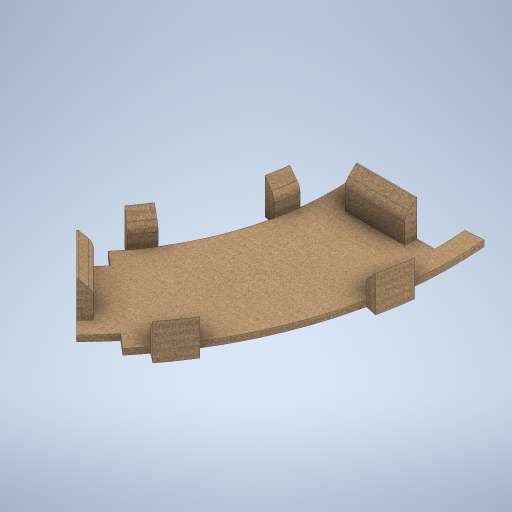
# Autodesk Inventor part: MC Plate
Saved by Autodesk Inventor 2023 (Build 270158000, 158)
## iProperties
Created: 2023-01-27
Part Number: MC Plate
Material: MDF Medium Density Fiberboard
Document SubType Name: Modeling
Designer: cheng
Density: 0.8 g/cm^3
Appearance: Cardboard - Corrugated
Mass: 204.328 g
Surface Area: 611.32 cm^2
Volume: 255.411 cm^3
Author: cheng
Autodesk Inventor part; units mm, degrees
ref_plane "YZ Plane" through (0, 0, 0) normal (1, 0, 0) x (0, 1, 0)
ref_plane "XZ Plane" through (0, 0, 0) normal (0, 1, 0) x (-1, 0, 0)
ref_plane "XY Plane" through (0, 0, 0) normal (0, 0, 1) x (1, 0, 0)
sketch "Sketch1" plane through (0, 0, 0) normal (0, 1, 0) x (-1, 0, 0)
  circle A0 centre (0, 0) radius 215
  circle A1 centre (0, 0) radius 315
  line L0 (0, 0) -> (-315, 0)
  line L1 (0, 0) -> (-222.7386, 222.7386)
  line L2 (0, 0) -> (-313.8013, -27.4541)
  line L3 (0, 0) -> (-241.304, 202.4781)
  circle A2 centre (0, 0) radius 230
  circle A3 centre (0, 0) radius 300
  point P0 (-152.028, 152.028)
  point P1 (-215, 0)
  point P2 (-212.132, 212.132)
  point P3 (-229.8133, 192.8363)
  point P4 (-298.8584, -26.1467)
  point P5 (-300, 0)
  point P6 (-230, 0)
  point P7 (-229.1248, -20.0458)
  point P8 (-214.1819, -18.7385)
  point P9 (-164.6996, 138.1993)
  point P10 (-176.1902, 147.8412)
  point P11 (-162.6346, 162.6346)
  dimension "d1" = 430
  dimension "d2" = 45
  dimension "d31" = 100
  dimension "d47" = 5
  dimension "d48" = 5
  dimension "d49" = 15
  dimension "d50" = 15
  constraints: 8 end point, 4 centre point, 4 coincident, 4 point on circle, 1 horizontal
  measures "d1" diameter of A0
  measures "d2" angle of L0 L1
  measures "d31" radial gap between concentric circles of A0 A1
  measures "d47" angle of L2 L0
  measures "d48" angle of L3 L1
  measures "d49" radial gap between concentric circles of A0 A2
  measures "d50" radial gap between concentric circles of A3 A1
extrude "Extrusion1" add sketch "Sketch1" along normal blind 5 contours L2 A2 L0 A0 | A0 L0 A2 L3 | A2 L3 A3 L1 | A2 L0 A3 L3 | L2 A1 L0 A3 | A3 L0 A1 L3
sketch "Sketch2" plane through (0, 0, 0) normal (0, 1, 0) x (1, 0, 0)
  circle A0 centre (0, 0) radius 205
  circle A1 centre (0, 0) radius 215
  circle A2 centre (0, 0) radius 315
  circle A3 centre (0, 0) radius 325
  line L0 (0, 0) -> (259.5565, -195.5899)
  line L1 (0, 0) -> (275.6156, -172.2238)
  line L2 (0, 0) -> (317.898, -67.5713)
  line L3 (0, 0) -> (322.5775, -39.6075)
  line L4 (300, 0) -> (230, 0) projected
  point P0 (315, 0)
  point P1 (215, 0)
  point P2 (312.652, -38.3888)
  point P3 (308.1165, -65.4922)
  point P4 (213.3974, -26.2019)
  point P5 (203.472, -24.9832)
  point P6 (200.5203, -42.6219)
  point P7 (210.3017, -44.701)
  point P8 (267.1352, -166.9246)
  point P9 (251.5702, -189.5717)
  point P10 (182.3303, -113.9326)
  point P11 (173.8499, -108.6334)
  point P12 (163.7203, -123.3721)
  point P13 (171.7066, -129.3902)
  dimension "d5" = 410
  dimension "d6" = 10
  dimension "d7" = 100
  dimension "d8" = 10
  dimension "d9" = 7
  dimension "d10" = 5
  dimension "d11" = 20
  dimension "d12" = 5
  constraints: 8 end point, 4 centre point, 4 coincident, 4 point on circle
  measures "d5" diameter of A0
  measures "d6" radial gap between concentric circles of A0 A1
  measures "d7" radial gap between concentric circles of A2 A1
  measures "d8" radial gap between concentric circles of A2 A3
  measures "d9" angle of L3 L4
  measures "d10" angle of L2 L3
  measures "d11" angle of L1 L2
  measures "d12" angle of L0 L1
extrude "Extrusion2" add sketch "Sketch2" along normal blind 30 contours A0 L1 A1 L0 | L3 A1 L2 A0 | A2 L1 A3 L0 | L3 A3 L2 A2
chamfer "Chamfer1" distance 10 angle 45 4 edges at (177.1871, 30, 121.7773) (259.5997, 30, 178.418) (212.0514, 30, 35.4852) (310.68, 30, 51.99)
sketch "Sketch3" plane through (0, 5, 0) normal (0, 1, 0) x (1, 0, 0)
  circle A0 centre (0, 0) radius 235
  circle A1 centre (0, 0) radius 285
  arc A2 (251.5702, -189.5717) -> (267.1352, -166.9246) centre (0, 0) ccw projected
  arc A3 (308.1165, -65.4922) -> (312.652, -38.3888) centre (0, 0) ccw projected
  arc A4 (241.304, -202.4781) -> (251.5702, -189.5717) centre (0, 0) ccw projected
  line L0 (300, 0) -> (230, 0) projected
  arc A5 (213.3974, -26.2019) -> (214.1819, 18.7385) centre (0, 0) ccw projected
  line L1 (162.6346, -162.6346) -> (212.132, -212.132) projected
  line L2 (166.1701, -166.1701) -> (201.5254, -201.5254)
  arc A6 (312.652, -38.3888) -> (313.8013, 27.4541) centre (0, 0) ccw projected
  arc A7 (267.1352, -166.9246) -> (308.1165, -65.4922) centre (0, 0) ccw projected
  arc A8 (171.7066, -129.3902) -> (182.3303, -113.9326) centre (0, 0) ccw projected
  arc A9 (164.6996, -138.1993) -> (171.7066, -129.3902) centre (0, 0) ccw projected
  arc A10 (210.3017, -44.701) -> (213.3974, -26.2019) centre (0, 0) ccw projected
  arc A11 (182.3303, -113.9326) -> (210.3017, -44.701) centre (0, 0) ccw projected
  line L3 (235, 0) -> (284.6303, 0)
  line L4 (284.8245, -10) -> (234.7871, -10)
  line L5 (208.4724, -194.3303) -> (173.0906, -158.9485)
  line L6 (229.8133, -192.8363) -> (241.304, -202.4781) projected
  line L7 (313.8013, 27.4541) -> (298.8584, 26.1467) projected
  arc A12 (300, 0) -> (298.8584, 26.1467) centre (0, 0) ccw projected
  arc A13 (230, 0) -> (229.1248, 20.0458) centre (0, 0) ccw projected
  line L8 (229.1248, 20.0458) -> (214.1819, 18.7385) projected
  line L9 (164.6996, -138.1993) -> (176.1902, -147.8412) projected
  arc A14 (162.6346, -162.6346) -> (176.1902, -147.8412) centre (0, 0) ccw projected
  arc A15 (212.132, -212.132) -> (229.8133, -192.8363) centre (0, 0) ccw projected
  point P0 (235, 0)
  point P1 (172.3223, -159.7812)
  point P2 (208.9866, -193.7772)
  point P3 (166.1701, -166.1701)
  point P4 (201.5254, -201.5254)
  point P5 (285, 0)
  point P6 (235, 0)
  point P7 (183.8478, -183.8478)
  point P8 (187.3833, -187.3833)
  dimension "d18" = 470
  dimension "d22" = 0
  dimension "d32" = 50
  dimension "d33" = 10
  dimension "d34" = 0
  dimension "d43" = 10
  constraints: 10 point on circle, 8 end point, 2 centre point, 2 coincident, 2 horizontal, 2 midpoint, 1 line through centre, 1 parallel
  measures "d18" diameter of A0
  measures "d22" distance between parallel lines of L1 L2
  measures "d32" radial gap between concentric circles of A1 A0
  measures "d33" distance between parallel lines of L3 L4
  measures "d34" distance between parallel lines of L0 L3
  measures "d43" distance between parallel lines of L5 L2
extrude "Extrusion3" add sketch "Sketch3" along normal blind 30 contours L0 A1 L4 A0 | A0 L5 A1 L1
chamfer "Chamfer3" distance 9 angle 45 2 edges at (259.8058, 35, 10) (190.7815, 35, 176.6394)
fillet "Fillet1" radius 10 6 edges at (259.8058, 26, 10) (310.68, 20.0005, 51.99) (259.5997, 20.0005, 178.418) (177.1871, 20.0005, 121.7773) (212.0514, 20.0005, 35.4852) (190.7815, 26, 176.6394)
sketch "Sketch4" plane through (0, 5, 0) normal (0, 1, 0) x (1, 0, 0)
  arc A0 (201.5254, -201.5254) -> (208.4724, -194.3303) centre (0, 0) ccw projected
  line L0 (201.5254, -201.5254) -> (212.132, -212.132) projected
  arc A1 (241.304, -202.4781) -> (251.5702, -189.5717) centre (0, 0) ccw projected
  arc A2 (251.5702, -189.5717) -> (267.1352, -166.9246) centre (0, 0) ccw projected
  arc A3 (267.1352, -166.9246) -> (308.1165, -65.4922) centre (0, 0) ccw projected
  arc A4 (308.1165, -65.4922) -> (312.652, -38.3888) centre (0, 0) ccw projected
  arc A5 (312.652, -38.3888) -> (313.8013, 27.4541) centre (0, 0) ccw projected
  line L1 (300, 0) -> (285, 0) projected
  arc A6 (284.8245, -10) -> (285, 0) centre (0, 0) ccw projected
  line L2 (284.8245, -10) -> (234.7871, -10) projected
  arc A7 (234.7871, -10) -> (235, 0) centre (0, 0) ccw projected
  line L3 (235, 0) -> (230, 0) projected
  arc A8 (213.3974, -26.2019) -> (214.1819, 18.7385) centre (0, 0) ccw projected
  arc A9 (210.3017, -44.701) -> (213.3974, -26.2019) centre (0, 0) ccw projected
  arc A10 (182.3303, -113.9326) -> (210.3017, -44.701) centre (0, 0) ccw projected
  arc A11 (171.7066, -129.3902) -> (182.3303, -113.9326) centre (0, 0) ccw projected
  arc A12 (164.6996, -138.1993) -> (171.7066, -129.3902) centre (0, 0) ccw projected
  line L4 (162.6346, -162.6346) -> (166.1701, -166.1701) projected
  arc A13 (166.1701, -166.1701) -> (173.0906, -158.9485) centre (0, 0) ccw projected
  line L5 (234.7871, -10) -> (214.7673, -10)
  arc A14 (213.3974, -26.2019) -> (214.1819, 18.7385) centre (0, 0) ccw projected
  line L6 (284.8245, -10) -> (314.8412, -10)
  line L7 (171.8681, -160.2696) -> (157.241, -146.6296)
  line L8 (208.4358, -194.3695) -> (230.3764, -214.8295)
  arc A15 (241.304, -202.4781) -> (251.5702, -189.5717) centre (0, 0) ccw projected
  line L9 (173.0906, -158.9485) -> (208.4724, -194.3303) projected
  arc A16 (230, 0) -> (229.1248, 20.0458) centre (0, 0) ccw projected
  line L10 (229.1248, 20.0458) -> (214.1819, 18.7385) projected
  line L11 (164.6996, -138.1993) -> (176.1902, -147.8412) projected
  arc A17 (162.6346, -162.6346) -> (176.1902, -147.8412) centre (0, 0) ccw projected
  arc A18 (212.132, -212.132) -> (229.8133, -192.8363) centre (0, 0) ccw projected
  line L12 (229.8133, -192.8363) -> (241.304, -202.4781) projected
  line L13 (313.8013, 27.4541) -> (298.8584, 26.1467) projected
  arc A19 (300, 0) -> (298.8584, 26.1467) centre (0, 0) ccw projected
  point P0 (222.7386, -222.7386)
  point P1 (215, 0)
  dimension "d39" = 43
  constraints: 8 end point, 4 point on circle, 2 line through centre, 2 point on line, 1 horizontal
  measures "d39" angle of L6 L7
sketch "Sketch5" plane through (0, 5, 0) normal (0, 1, 0) x (1, 0, 0)
  arc A0 (234.7871, -10) -> (235, 0) centre (0, 0) ccw projected
  line L0 (235, 0) -> (230, 0) projected
  arc A1 (213.3974, -26.2019) -> (214.1819, 18.7385) centre (0, 0) ccw projected
  arc A2 (210.3017, -44.701) -> (213.3974, -26.2019) centre (0, 0) ccw projected
  arc A3 (182.3303, -113.9326) -> (210.3017, -44.701) centre (0, 0) ccw projected
  arc A4 (171.7066, -129.3902) -> (182.3303, -113.9326) centre (0, 0) ccw projected
  arc A5 (164.6996, -138.1993) -> (171.7066, -129.3902) centre (0, 0) ccw projected
  line L1 (162.6346, -162.6346) -> (166.1701, -166.1701) projected
  arc A6 (166.1701, -166.1701) -> (173.0906, -158.9485) centre (0, 0) ccw projected
  line L2 (173.0906, -158.9485) -> (208.4724, -194.3303) projected
  arc A7 (201.5254, -201.5254) -> (208.4724, -194.3303) centre (0, 0) ccw projected
  line L3 (201.5254, -201.5254) -> (212.132, -212.132) projected
  arc A8 (241.304, -202.4781) -> (251.5702, -189.5717) centre (0, 0) ccw projected
  arc A9 (251.5702, -189.5717) -> (267.1352, -166.9246) centre (0, 0) ccw projected
  arc A10 (267.1352, -166.9246) -> (308.1165, -65.4922) centre (0, 0) ccw projected
  arc A11 (308.1165, -65.4922) -> (312.652, -38.3888) centre (0, 0) ccw projected
  arc A12 (312.652, -38.3888) -> (313.8013, 27.4541) centre (0, 0) ccw projected
  line L4 (300, 0) -> (285, 0) projected
  arc A13 (284.8245, -10) -> (285, 0) centre (0, 0) ccw projected
  line L5 (284.8245, -10) -> (234.7871, -10) projected
  line L6 (222.7386, -222.7386) -> (0, 0) construction
  line L7 (0, 0) -> (315, 0) construction
  circle A14 centre (0, 0) radius 215
  circle A15 centre (0, 0) radius 315
  arc A16 (230, 0) -> (229.1248, 20.0458) centre (0, 0) ccw projected
  line L8 (229.1248, 20.0458) -> (214.1819, 18.7385) projected
  line L9 (164.6996, -138.1993) -> (176.1902, -147.8412) projected
  arc A17 (162.6346, -162.6346) -> (176.1902, -147.8412) centre (0, 0) ccw projected
  arc A18 (212.132, -212.132) -> (229.8133, -192.8363) centre (0, 0) ccw projected
  line L10 (229.8133, -192.8363) -> (241.304, -202.4781) projected
  line L11 (313.8013, 27.4541) -> (298.8584, 26.1467) projected
  arc A19 (300, 0) -> (298.8584, 26.1467) centre (0, 0) ccw projected
  dimension "d44" = 45
  dimension "d45" = 630
  dimension "d46" = 430
  constraints: 4 end point, 2 centre point, 2 coincident, 1 collinear, 1 concentric, 1 horizontal
  measures "d44" angle of L7 L6
  measures "d45" diameter of A15
  measures "d46" diameter of A14
body "Solid1"
